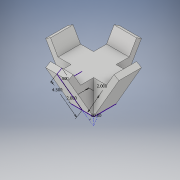
# Autodesk Inventor part: 4-Tool_Head
Saved by Autodesk Inventor 2019 (Build 230136000, 136)
## iProperties
Created: 2021-01-21
Part Number: 4-Tool_Head
Material: Generic
Document SubType Name: Modeling
Designer: zhanb
Density: 1 g/cm^3
Appearance: Default
Author: zhanb
Autodesk Inventor part; units mm, degrees
ref_plane "YZ Plane" through (0, 0, 0) normal (1, 0, 0) x (0, 1, 0)
ref_plane "XZ Plane" through (0, 0, 0) normal (0, 1, 0) x (-1, 0, 0)
ref_plane "XY Plane" through (0, 0, 0) normal (0, 0, 1) x (1, 0, 0)
sketch "Sketch1" plane through (0, 0, 0) normal (0, 1, 0) x (-1, 0, 0)
  circle A0 centre (0, 0) radius 25.4 construction
  line L0 (-25.4, -25.4) -> (25.4, -25.4)
  line L1 (25.4, -25.4) -> (25.4, 25.4)
  line L2 (25.4, 25.4) -> (-25.4, 25.4)
  line L3 (-25.4, 25.4) -> (-25.4, -25.4)
  line L4 (-25.4, -25.4) -> (25.4, 25.4) construction
  line L5 (25.4, -25.4) -> (-25.4, 25.4) construction
  dimension "d0" = 50.8
  dimension "d1" = 50.8
  constraints: 12 end point, 2 midpoint, 2 parallel, 2 perpendicular, 1 centre point, 1 coincident, 1 horizontal
  measures "d0" distance of L0.end L1.end
  measures "d1" diameter of A0
extrude "Extrusion1" add sketch "Sketch1" along normal blind 76.2
sketch "Sketch3" plane through (0, 0, 0) normal (1, 0, 0) x (0, 1, 0)
  line L0 (-43.9941, 0) -> (0, 25.4) construction
  line L1 (0, -25.4) -> (0, 25.4) construction
  line L2 (76.2, 25.4) -> (0, 25.4) construction
  line L3 (0, 25.4) -> (0, 0) construction
  line L4 (-43.9941, 0) -> (0, 0) construction
  line L5 (-43.9941, 0) -> (0, -25.4) construction
  line L6 (98.9867, 82.55) -> (105.3367, 71.5515)
  line L7 (105.3367, 71.5515) -> (76.2, 54.7294)
  line L8 (76.2, 54.7294) -> (76.2, 25.4)
  line L9 (0, 25.4) -> (98.9867, 82.55)
  line L10 (0, 25.4) -> (76.2, 25.4)
  dimension "d14" = 60
  dimension "d15" = 12.7
  dimension "d16" = 114.3
  constraints: 20 end point, 3 perpendicular, 1 collinear, 1 midpoint, 1 parallel, 1 vertical, 1 other
  measures "d14" angle of L5 L0
  measures "d15" distance between parallel lines of L0 L7
  measures "d16" distance from line of L6 L0.end
extrude "Extrusion2" add sketch "Sketch3" along normal mid plane 50.8
pattern_circular "Circular Pattern1" count 4 over 360 about axis through (0, -10, 0) along (0, 1, 0) of "Extrusion2"
body "Solid1"
